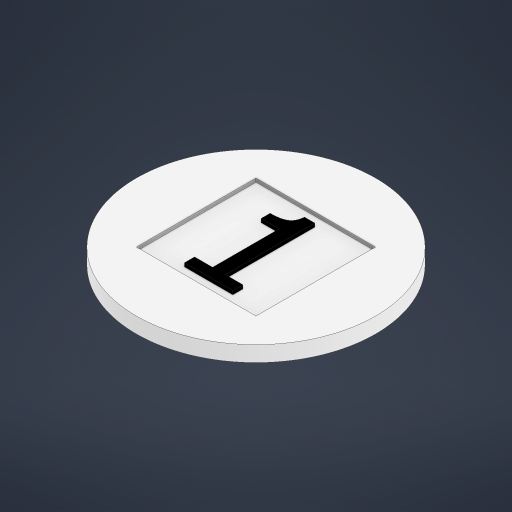
# Autodesk Inventor part: TopMarker1
Saved by Autodesk Inventor 2023 (Build 270158000, 158)
## iProperties
Created: 2023-03-04
Part Number: TopMarker1
Material: Generic
Document SubType Name: Modeling
Designer: Elias Braun
Density: 1 g/cm^3
Appearance: Default
Author: Elias Braun
Autodesk Inventor part; units mm, degrees
ref_plane "YZ Plane" through (0, 0, 0) normal (1, 0, 0) x (0, 1, 0)
ref_plane "XZ Plane" through (0, 0, 0) normal (0, 1, 0) x (-1, 0, 0)
ref_plane "XY Plane" through (0, 0, 0) normal (0, 0, 1) x (1, 0, 0)
sketch "Sketch1" plane through (0, 0, 0) normal (0, 1, 0) x (-1, 0, 0)
  circle A0 centre (0, 0) radius 20
  dimension "d0" = 40
  constraints: 1 centre point, 1 coincident
  measures "d0" diameter of A0
extrude "Extrusion1" add sketch "Sketch1" along normal blind 2.6
sketch "Sketch2" plane through (0, 2.6, 0) normal (0, 1, 0) x (1, 0, 0)
  line L0 (10, -10) -> (-10, -10)
  line L1 (-10, -10) -> (-10, 10)
  line L2 (-10, 10) -> (10, 10)
  line L3 (10, 10) -> (10, -10)
  line L4 (10, -10) -> (-10, 10) construction
  line L5 (-10, -10) -> (10, 10) construction
  point P0 (0, 0)
  dimension "d3" = 20
  dimension "d4" = 20
  constraints: 12 end point, 2 midpoint, 2 parallel, 1 horizontal, 1 perpendicular
  measures "d3" distance of L0.start L0.end
  measures "d4" distance of L0.end L1.end
extrude "Extrusion2" cut sketch "Sketch2" against normal blind 0.6
sketch "Sketch3" plane through (0, 2, 0) normal (0, 1, 0) x (1, 0, 0)
  line L0 (-6.2284, 8.396) -> (6.2284, 8.396) construction
  line L1 (6.2284, 8.396) -> (6.2284, -8.2578) construction
  line L2 (6.2284, -8.2578) -> (-6.2284, -8.2578) construction
  line L3 (-6.2284, -8.2578) -> (-6.2284, 8.396) construction
  line L4 (4.3854, -8.2578) -> (-3.7128, -8.2578)
  line L5 (-3.7128, -8.2578) -> (-3.7128, -6.5629)
  line L6 (-3.7128, -6.5629) -> (-0.6995, -6.5629)
  line L7 (-0.6995, -6.5629) -> (-0.6995, 4.5621)
  line L8 (-0.6995, 4.5621) -> (-3.7128, 4.5621)
  line L9 (-3.7128, 4.5621) -> (-3.7128, 6.0822)
  spline S0 degree 2 poles (-3.7128, 6.0822) (-2.0044, 6.0822) (-0.3901, 7.0508) (-0.2825, 8.396) knots 0 0 0 1 2 2 2
  line L10 (-0.2825, 8.396) -> (1.4394, 8.396)
  line L11 (1.4394, 8.396) -> (1.4394, -6.5629)
  line L12 (1.4394, -6.5629) -> (4.3854, -6.5629)
  line L13 (4.3854, -6.5629) -> (4.3854, -8.2578)
  point P0 (0, 0)
  point P1 (0, 0)
  constraints: 1 coincident, 2 other
extrude "Extrusion3" add sketch "Sketch3" along normal blind 0.6
body "Solid1"
